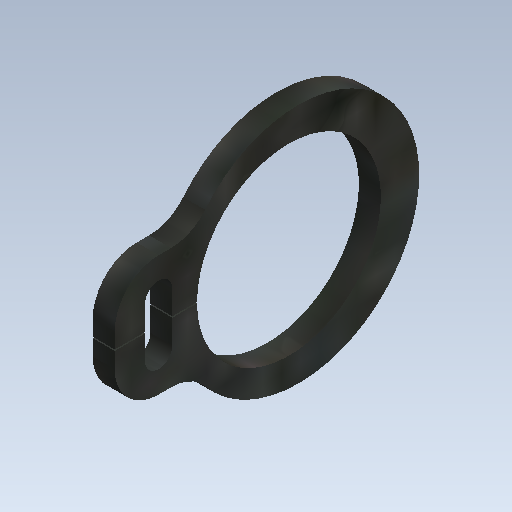
# Autodesk Inventor part: STWN7
Saved by Autodesk Inventor 2021 (Build 250183000, 183)
## iProperties
Part Number: STWN7
Material: Steel
Catalog Web Link: www.cadenas.de
Description: STWN, STWS-Retaining Rings - C - External
Vendor: MISUMI
Document SubType Name: Modeling
Designer: partserver
Manufacturer: MISUMI
Mass: 0.206807 g
Surface Area: 1.164 cm^2
Volume: 0.0263448 cm^3
Density: 7.85 g/cm^3
Appearance: Plate
Category: PARTsolutions
Company: MISUMI
PSOL_IDENT_0: {$CADENAS_DATA\23d-libs\misumi\metric\28_keys_magnets\stwn.prj},157 {VTYP=3D},{NB=STWN7},{LINA=STWN7
PSOL_IDENT_1: },{NN=STWN, STWS},{DATE=09.09.2019 15:27:57},{GEOMDATE=19.07.2012 00:00:00},{VERSION=},{LINEID=50},{
PSOL_IDENT_2: WBVAR=MAT},{WBNUMERIC=}  {NB=STWN7},{LINA=STWN7},{KT=DUMMY},{PN=STWN7},{TYPE=STWN},{MAT=1},{HARD=44~
PSOL_IDENT_3: 53HRC},{NO=7},{MATALG='1','Spring Steel','2','304 Stainless Steel-CSP'},{DD3=6.5},{DD3TOL=+0.06/-0.2
PSOL_IDENT_4: },{TT=0.80},{TTTOL=+0.04/-0.04},{BB=1.4},{AA=3.0},{DD0=1.0},{DD4=14.0},{DD1=7},{DD2=6.70},{DD2TOL=0/
PSOL_IDENT_5: -0.06},{MM=0.90},{MMTOL=+0.10/0},{NN=0.5},{H1=1.6},{A3=0.05},{A2=1.80},{A1=4.40},{R2=1.60},{R1=1.60}
NB: STWN7
NN: 0.5
NT: Retaining Rings - C - External
NBSYN: $PN.
LINA: STWN7
CATALOG: Misumi
PN: STWN7
MAT: Spring Steel
HARD: 44~53HRC
NO: 7
DD3: 6.5
DD3TOL: +0.06/-0.2
TT: 0.8
TTTOL: +0.04/-0.04
BB: 1.4
AA: 3
DD0: 1
DD4: 14
DD1: 7
DD2: 6.7
DD2TOL: 0/-0.06
MM: 0.9
MMTOL: +0.10/0
SUPPLIER: MISUMI
ARTICLENO: STWN7
BOMINFO: STWN7
CREATOR: CADENAS GmbH
Title: STWN7
Author: Cadenas PARTsolutions
Comments: Retaining Rings - C - External
Autodesk Inventor part; units mm, degrees
sketch "Sketch_5" plane through (0, 0, 0) normal (1, 0, 0) x (0, 1, 0)
  arc A0 (-3.0551, -2.7867) -> (-3.0551, 2.7867) centre (0.35, 0) ccw
  arc A1 (-4.2933, 2.2) -> (-3.0551, 2.7867) centre (-4.2933, 3.8) ccw
  line L0 (-4.2933, 2.2) -> (-4.75, 2.2)
  arc A2 (-4.75, 2.2) -> (-6.35, 0.6) centre (-4.75, 0.6) ccw
  line L1 (-6.35, 0.6) -> (-6.35, 0.025)
  line L2 (-6.35, 0.025) -> (-5.25, 0.025)
  line L3 (-5.25, 0.025) -> (-5.25, 0.9)
  arc A3 (-4.25, 0.9) -> (-5.25, 0.9) centre (-4.75, 0.9) ccw
  line L4 (-4.25, 0.9) -> (-4.25, 0.025)
  line L5 (-4.25, 0.025) -> (-3.3499, 0.025)
  arc A4 (-3.3499, -0.025) -> (-3.3499, 0.025) centre (0, 0) ccw
  line L6 (-3.3499, -0.025) -> (-4.25, -0.025)
  line L7 (-4.25, -0.025) -> (-4.25, -0.9)
  arc A5 (-5.25, -0.9) -> (-4.25, -0.9) centre (-4.75, -0.9) ccw
  line L8 (-5.25, -0.9) -> (-5.25, -0.025)
  line L9 (-5.25, -0.025) -> (-6.35, -0.025)
  line L10 (-6.35, -0.025) -> (-6.35, -0.6)
  arc A6 (-6.35, -0.6) -> (-4.75, -2.2) centre (-4.75, -0.6) ccw
  line L11 (-4.75, -2.2) -> (-4.2933, -2.2)
  arc A7 (-3.0551, -2.7867) -> (-4.2933, -2.2) centre (-4.2933, -3.8) ccw
  constraints: 24 end point, 16 point on circle, 8 centre point
extrude "Extrusion1" add sketch "Sketch_5" along normal mid plane 0.8
ref_plane "1_XY" through (0, 0, 0) normal (1, 0, 0) x (0, 0, -1)
ref_plane "1_YZ" through (0, 0, 0) normal (0, 0, -1) x (0, 1, 0)
ref_plane "1_ZX" through (0, 0, 0) normal (0, 1, 0) x (1, 0, 0)
ref_plane "combination_module_XY" through (0.4, 0, 0) normal (1, 0, 0) x (0, 0, -1)
ref_plane "combination_module_YZ" through (0.4, 0, 0) normal (0, 0, -1) x (0, 1, 0)
ref_plane "combination_module_ZX" through (0.4, 0, 0) normal (0, 1, 0) x (1, 0, 0)
body "Solid1"
